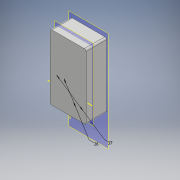
# Autodesk Inventor part: NespressoSpeedfiller-base
Saved by Autodesk Inventor 2017 (Build 210142000, 142)
## iProperties
Created: 2018-08-27
Part Number: NespressoSpeedfiller-base
Material: Generic
Document SubType Name: Modeling
Designer: 45027374
Density: 1 g/cm^3
Appearance: Default
Author: 45027374
Autodesk Inventor part; units mm, degrees
ref_plane "YZ Plane" through (0, 0, 0) normal (1, 0, 0) x (0, 1, 0)
ref_plane "XY Plane" through (0, 0, 0) normal (0, 0, 1) x (1, 0, 0)
sketch "Sketch1" plane through (0, 0, 0) normal (0, 1, 0) x (-1, 0, 0)
  line L0 (25.9, 0) -> (-25.9, 0) projected
  line L1 (0, -25.9) -> (0, 25.9) projected
  circle A0 centre (0, 0) radius 18.5 construction
  circle A1 centre (0, 0) radius 13 construction
  dimension "d0" = 37
  dimension "d1" = 26
  constraints: 2 centre point, 2 coincident
  measures "d0" diameter of A0
  measures "d1" diameter of A1
sketch "Sketch2" plane through (0, 0, 0) normal (0, 1, 0) x (-1, 0, 0)
  line L0 (29.4, 0) -> (-29.4, 0) projected
  line L1 (0, -36.3) -> (0, 70.8) projected
  line L2 (-21, 55.5) -> (-21, -21)
  line L3 (-21, -21) -> (21, -21)
  line L4 (21, -21) -> (21, 55.5)
  line L5 (-21, 55.5) -> (21, 55.5)
  point P0 (0, 0)
  dimension "d3" = 42
  dimension "d29" = 21
  dimension "d30" = 55.5
  constraints: 8 end point, 1 horizontal, 1 parallel, 1 other
  measures "d3" distance of L2.end L3.end
  measures "d29" distance between parallel lines of L0 L3
  measures "d30" distance between parallel lines of L5 L0
extrude "Extrusion1" add sketch "Sketch2" along normal blind 22
sketch "Sketch8" plane through (0, 0, 0) normal (0, 1, 0) x (-1, 0, 0)
  circle A0 centre (0, 0) radius 12.25
  dimension "d34" = 24.5
  constraints: 1 centre point, 1 coincident
  measures "d34" diameter of A0
sketch "Sketch9" plane through (0, 22, 0) normal (0, 1, 0) x (1, 0, 0)
  circle A0 centre (0, 0) radius 13
  circle A1 centre (0, 0) radius 15
  dimension "d40" = 26
  dimension "d41" = 30
  constraints: 2 centre point, 2 coincident
  measures "d40" diameter of A0
  measures "d41" diameter of A1
extrude "Extrusion10" [suppressed]
sketch "Sketch10" plane through (0, 5, 0) normal (0, 1, 0) x (1, 0, 0)
  arc A0 (16, 0) -> (-16, 0) centre (0, 0) ccw projected
  line L0 (1.5, -18) -> (-1.5, -18)
  line L1 (-29.4, 0) -> (29.4, 0) projected
  line L2 (0, 36.3) -> (0, -70.8) projected
  line L3 (1.5, -12) -> (-1.5, -12)
  line L4 (1.5, -12) -> (1.5, -18)
  line L5 (-1.5, -18) -> (-1.5, -12)
  dimension "d48" = 3
  dimension "d49" = 12
  dimension "d50" = 6
  constraints: 8 end point, 2 perpendicular, 1 horizontal, 1 parallel, 1 other
  measures "d48" distance between parallel lines of L4 L5
  measures "d49" distance between parallel lines of L1 L3
  measures "d50" distance between parallel lines of L0 L3
extrude "Extrusion11" [suppressed]
ref_plane "Work Plane1" through (0, 5, 0) normal (0, 1, 0) x (-1, 0, 0)
fillet "Fillet3" radius 2 2 edges at (21, 11, 55.5) (-21, 11, 55.5)
ref_plane "Work Plane2" through (0, 22, 0) normal (0, 1, 0) x (-1, 0, 0)
sketch "Sketch16" plane through (0, 22, 0) normal (0, 1, 0) x (-1, 0, 0)
  line L0 (29.4, 0) -> (-29.4, 0) projected
  line L1 (0, -72.3) -> (0, 76.8) projected
  circle A0 centre (0, 0) radius 13.75
  dimension "d97" = 27.5
  constraints: 1 centre point, 1 coincident
  measures "d97" diameter of A0
loft "Loft1" cut profiles "Sketch8", "Sketch16"
pattern_linear "Rectangular Pattern2" count 2 spacing 37 along (0, 0, 1) of "Loft1"
sketch "Sketch17" plane through (0, 0, 0) normal (0, 1, 0) x (-1, 0, 0)
  line L0 (-21, 55.5) -> (21, 55.5)
  line L1 (21, 55.5) -> (21, -21)
  line L2 (21, -21) -> (-21, -21)
  line L3 (-21, -21) -> (-21, 55.5)
  line L4 (29.4, 0) -> (-29.4, 0) projected
  line L5 (0, -72.3) -> (0, 76.8) projected
  point P0 (0, 0)
  dimension "d105" = 21
  dimension "d106" = 55.5
  dimension "d107" = 42
  constraints: 8 end point, 2 parallel, 1 horizontal, 1 perpendicular, 1 other
  measures "d105" distance between parallel lines of L2 L4
  measures "d106" distance between parallel lines of L0 L4
  measures "d107" distance between parallel lines of L1 L3
extrude "Extrusion18" add sketch "Sketch17" against normal blind 2
fillet "Fillet8" radius 2 2 edges at (21, -1, 55.5) (-21, -1, 55.5)
sketch "Sketch18" plane through (0, 0, 0) normal (1, 0, 0) x (0, 1, 0)
  line L0 (22, -21) -> (0, -21)
  line L1 (0, -21) -> (0, -51)
  line L2 (0, -51) -> (22, -51)
  line L3 (22, -51) -> (22, -21)
  line L4 (20, -23) -> (2, -23)
  line L5 (2, -23) -> (2, -49)
  line L6 (2, -49) -> (20, -49)
  line L7 (20, -49) -> (20, -23)
  line L8 (-7.4, 0) -> (26.9, 0) projected
  line L9 (0, -72.3) -> (0, 76.8) projected
  point P0 (0, 0)
  dimension "d119" = 21
  dimension "d120" = 51
  dimension "d121" = 22
  dimension "d122" = 2
  dimension "d123" = 23
  dimension "d124" = 20
  dimension "d125" = 49
  constraints: 16 end point, 4 parallel, 2 horizontal, 2 perpendicular, 1 collinear
  measures "d119" distance between parallel lines of L8 L0
  measures "d120" distance between parallel lines of L8 L2
  measures "d121" distance between parallel lines of L3 L1
  measures "d122" distance between parallel lines of L9 L5
  measures "d123" distance between parallel lines of L8 L4
  measures "d124" distance between parallel lines of L1 L7
  measures "d125" distance between parallel lines of L8 L6
extrude "Extrusion20" [suppressed]
fillet "Fillet10" [suppressed]
fillet "Fillet11" radius 2 2 edges at (21, 10, -21) (-21, 10, -21)
sketch "Sketch19" plane through (0, 22, 0) normal (0, 1, 0) x (-1, 0, 0)
  line L0 (-40.8821, 18.5) -> (60.1438, 18.5) construction
  line L1 (0, -36.3) -> (0, 70.8) construction
  line L2 (0, -36.3) -> (0, 70.8) construction
  line L3 (80.349, 0) -> (-61.0873, 0) construction
  arc A0 (15.5, 23.5) -> (15.5, 13.5) centre (15.5, 18.5) ccw
  line L4 (15.5, 23.5) -> (15.5, 13.5)
  arc A1 (-15.5, 13.5) -> (-15.5, 23.5) centre (-15.5, 18.5) ccw
  line L5 (-15.5, 23.5) -> (-15.5, 13.5)
  point P0 (0, 0)
  dimension "d130" = 18.5
  dimension "d131" = 15.5
  dimension "d132" = 10
  dimension "d133" = 15.5
  constraints: 6 end point, 4 point on circle, 3 symmetric about line, 2 centre point, 1 horizontal, 1 parallel, 1 point on line, 1 other
  measures "d130" distance between parallel lines of L3 L0
  measures "d131" distance from line of L1 A0.centre
  measures "d132" diameter of A0
  measures "d133" distance between parallel lines of L1 L4
extrude "Extrusion21" add sketch "Sketch19" along normal blind 5
fillet "Fillet12" radius 1 4 edges at (15.5, 24.5, 13.5) (15.5, 24.5, 23.5) (-15.5, 24.5, 23.5) (-15.5, 24.5, 13.5)
body "Solid1"
